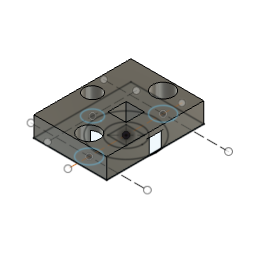
on_off_block v3 (Autodesk Fusion 360 design; units mm, degrees)
Autodesk Fusion 360 part; units mm, degrees
note: some values were not read from the file. Set by a fixed rule: which sketch regions a step uses.
sketch "Skizze1" plane through (0, 0, 0) normal (0, 0, 1) x (1, 0, 0)
  line L0 (-18, 20) -> (12, 20)
  line L1 (12, 20) -> (12, -20)
  line L2 (12, -20) -> (-18, -20)
  line L3 (-18, -20) -> (-18, 20)
  line L4 (0, 23) -> (0, -24) construction
  line L5 (-24.4424, 15.24) -> (27, 15.24) construction
  line L6 (-24, -15.24) -> (24, -15.24) construction
  line L7 (-13.79, 18) -> (-13.79, -18.6195) construction
  circle A0 centre (0, 15.24) radius 4.25
  circle A1 centre (0, -15.24) radius 4.25
  circle A2 centre (-13.79, -0.0668) radius 3.5
  circle A3 centre (0, 0) radius 12.25
  line L8 (3.75, -3.75) -> (-3.75, -3.75)
  line L9 (-3.75, -3.75) -> (-3.75, 3.75)
  line L10 (-3.75, 3.75) -> (3.75, 3.75)
  line L11 (3.75, 3.75) -> (3.75, -3.75)
  line L12 (3.75, -3.75) -> (-3.75, 3.75) construction
  line L13 (-3.75, -3.75) -> (3.75, 3.75) construction
  circle A4 centre (0, 0) radius 6.65
  dimension "d1" = 12
  dimension "d2" = 18
  dimension "d3" = 20
  dimension "d4" = 20
  dimension "d5" = 15.24
  dimension "d6" = 15.24
  dimension "d7" = 13.79
  dimension "d8" = 8.5
  dimension "d9" = 8.5
  dimension "d10" = 7
  dimension "d11" = 24.5
  dimension "d12" = 7.5
  dimension "d13" = 7.5
  dimension "d24" = 4.76
  dimension "d25" = 13.3
  constraint horizontal L0
  constraint vertical L1
  constraint horizontal L2
  constraint vertical L3
  constraint perpendicular L0 L4
  constraint perpendicular L3 L5
  constraint perpendicular L3 L6
  constraint perpendicular L6 L7
  constraint coincident L4 A0.centre
  constraint coincident L5 A0.centre
  constraint midpoint L6 A1.centre
  constraint coincident L7 A2.centre
  constraint coincident A3.centre A4.centre
  constraint horizontal L8
  constraint perpendicular L8 L9
  constraint parallel L8 L10
  constraint parallel L9 L11
  constraint coincident L12 A3.centre
  constraint coincident L13 A3.centre
  constraint concentric A3 A4
  measures "d1" distance of A3.centre L1
  measures "d2" distance of A3.centre L3
  measures "d3" distance of A3.centre L0
  measures "d4" distance of A3.centre L2
  measures "d5" distance of A3.centre L5
  measures "d6" distance of A3.centre L6
  measures "d7" distance of A3.centre L7
  measures "d8" diameter of A0
  measures "d9" diameter of A1
  measures "d10" diameter of A2
  measures "d11" diameter of A3
  measures "d12" distance of L8 L10
  measures "d13" distance of L9 L11
  measures "d24" distance of L0 L5
  measures "d25" diameter of A4
extrude "Extrusion1" add sketch "Skizze1" along normal blind 8.3 contours L0 L1 L2 L3 A0 A1 A2 A3 | L1 A0 A1 A2 A3 | A0 A3 | A0 A3 | A1 A3 | A1 A3 | A2 A3 | A2 A3 | L8 L9 L10 L11 | A4
extrude "Extrusion6" cut sketch "Skizze1" along normal blind 10 contours A0 A3 | A0 A3 | A1 A3 | A1 A3 | A2 A3 | A2 A3 | L8 L9 L10 L11
extrude "Extrusion7" cut sketch "Skizze1" along normal blind 6.3 contours L1 A0 A1 A2 A3
extrude "Extrusion8" add sketch "Skizze1" against normal blind 1.4 contours A4
